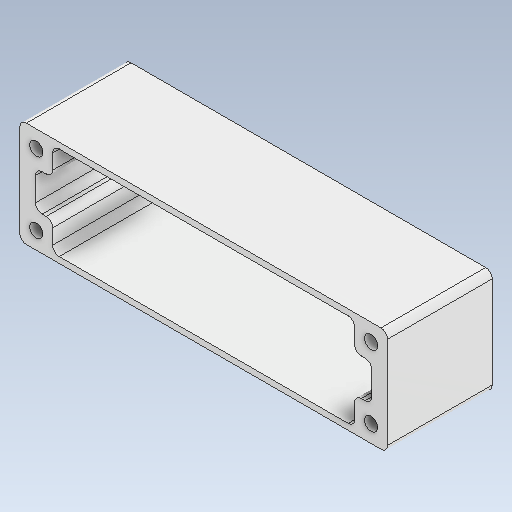
# Autodesk Inventor part: Battery Holder
Saved by Autodesk Inventor 2020 (Build 240168000, 168)
## iProperties
Created: 2020-02-03
Part Number: Battery Holder
Material: PC/ABS Plastic
Document SubType Name: Modeling
Designer: GJCla
Density: 0.357273 g/cm^3
Appearance: Smooth - White
Author: GJCla
Autodesk Inventor part; units mm, degrees
ref_plane "YZ Plane" through (0, 0, 0) normal (1, 0, 0) x (0, 1, 0)
ref_plane "XZ Plane" through (0, 0, 0) normal (0, 1, 0) x (-1, 0, 0)
sketch "Sketch1" plane through (0, 0, 0) normal (0, 0, 1) x (1, 0, 0)
  arc A0 (68.5, 19.5) -> (65.5, 22.5) centre (65.5, 19.5) ccw projected
  line L0 (-65.5, 22.5) -> (65.5, 22.5) projected
  arc A1 (-65.5, 22.5) -> (-68.5, 19.5) centre (-65.5, 19.5) ccw projected
  line L1 (-68.5, -19.5) -> (-68.5, 19.5) projected
  arc A2 (-68.5, -19.5) -> (-65.5, -22.5) centre (-65.5, -19.5) ccw projected
  line L2 (65.5, -22.5) -> (-65.5, -22.5) projected
  arc A3 (65.5, -22.5) -> (68.5, -19.5) centre (65.5, -19.5) ccw projected
  line L3 (68.5, 19.5) -> (68.5, -19.5) projected
  line L4 (88.6498, -25.3956) -> (-89.1502, -25.3956)
  line L5 (-89.1502, -25.3956) -> (-89.1502, 25.4044)
  line L6 (-89.1502, 25.4044) -> (88.6498, 25.4044)
  line L7 (88.6498, 25.4044) -> (88.6498, -25.3956)
  line L8 (-0.2502, 266.6127) -> (-0.2502, -243.9407)
  point P0 (0, 0)
  dimension "d23" = 177.8
  dimension "d24" = 50.8
  constraints: 10 end point, 2 horizontal, 2 parallel, 1 perpendicular, 1 vertical, 3 other
  measures "d23" distance of L5.end L6.end
  measures "d24" distance of L4.end L5.end
ref_plane "Work Plane1" through (-104.8982, -25.3956, -49) normal (0, 0, 1) x (1, 0, 0)
extrude "Extrusion1" add sketch "Sketch1" against normal up to surface (49 mm away) contours A0 L0 L8 L6 L7 L4 L2 A3 L3 | L0 A1 L1 A2 L2 L8 L4 L5 L6
sketch "Sketch2" plane through (0, 0, 0) normal (0, 0, 1) x (1, 0, 0)
  line L0 (88.6498, -25.3956) -> (88.6498, 25.4044) projected
  line L1 (-89.1502, 25.4044) -> (-89.1502, -25.3956) projected
  arc A0 (68.5, 19.5) -> (65.5, 22.5) centre (65.5, 19.5) ccw projected
  line L2 (68.5, 19.5) -> (68.5, -19.5) projected
  arc A1 (65.5, -22.5) -> (68.5, -19.5) centre (65.5, -19.5) ccw projected
  line L3 (65.5, -22.5) -> (-65.5, -22.5) projected
  arc A2 (-68.5, -19.5) -> (-65.5, -22.5) centre (-65.5, -19.5) ccw projected
  line L4 (-68.5, -19.5) -> (-68.5, 19.5) projected
  arc A3 (-65.5, 22.5) -> (-68.5, 19.5) centre (-65.5, 19.5) ccw projected
  line L5 (-65.5, 22.5) -> (65.5, 22.5) projected
  line L6 (65.5, 22.5) -> (-65.5, 22.5) projected
  line L7 (-65.5, 22.5) -> (-73.2752, 22.5)
  line L8 (-73.2752, 22.5) -> (-73.2752, 8.8856)
  line L9 (-73.2752, 8.8856) -> (-81.5302, 8.8856)
  line L10 (-81.5302, 8.8856) -> (-81.5302, -8.8944)
  line L11 (-81.5302, -8.8944) -> (-73.2752, -8.8944)
  line L12 (-73.2752, -8.8944) -> (-73.2752, -22.5088)
  line L13 (-73.2752, -22.5088) -> (72.7748, -22.5088)
  line L14 (72.7748, -22.5088) -> (72.7748, -8.8944)
  line L15 (72.7748, -8.8944) -> (81.0298, -8.8944)
  line L16 (81.0298, -8.8944) -> (81.0298, 8.8856)
  line L17 (81.0298, 8.8856) -> (72.7748, 8.8856)
  line L18 (72.7748, 8.8856) -> (72.7748, 22.5)
  line L19 (-65.5, 22.5) -> (72.7748, 22.5)
  line L20 (88.6498, 25.4044) -> (-89.1502, 25.4044) projected
  line L21 (-89.1502, -25.3956) -> (88.6498, -25.3956) projected
  point P0 (0, 0)
  dimension "d4" = 45.0088
  dimension "d5" = 17.78
  dimension "d6" = 7.62
  dimension "d7" = 7.62
  dimension "d8" = 146.05
  constraints: 26 end point, 8 perpendicular, 7 point on line, 3 collinear, 1 horizontal
  measures "d4" distance between parallel lines of L13 L6
  measures "d5" distance between parallel lines of L9 L11
  measures "d6" distance between parallel lines of L1 L10
  measures "d7" distance between parallel lines of L0 L16
  measures "d8" distance between parallel lines of L18 L8
extrude "Extrusion2" cut sketch "Sketch2" against normal up to next contours A0 L19 L18 L17 L16 L15 L14 L13 L12 L11 L10 L9 L8 L7 A3 L4 A2 L3 A1 L2
sketch "Sketch5" plane through (88.6498, 25.4044, -49) normal (0, 0, -1) x (-1, 0, 0)
  line L0 (0, 0) -> (0, -50.8) projected
  line L1 (177.8, -50.8) -> (0, -50.8) projected
  line L2 (0, 0) -> (177.8, 0)
  line L3 (177.8, 0) -> (177.8, -50.8)
  line L4 (177.8, -50.8) -> (0, -50.8)
  line L5 (0, -50.8) -> (0, 0)
  point P0 (88.6498, -25.4044)
  constraints: 8 end point, 2 parallel, 1 horizontal, 1 perpendicular
fillet "Fillet2" radius 3.175 12 edges at (-73.2752, 8.8856, -24.5) (-73.2752, 22.5, -24.5) (-81.5302, 8.8856, -24.5) (-81.5302, -8.8944, -24.5) (-73.2752, -8.8944, -24.5) (-73.2752, -22.5088, -24.5) (72.7748, -22.5088, -24.5) (72.7748, -8.8944, -24.5) (81.0298, -8.8944, -24.5) (81.0298, 8.8856, -24.5) (72.7748, 8.8856, -24.5) (72.7748, 22.5, -24.5)
sketch "Sketch6" plane through (0, 0, 0) normal (0, 0, 1) x (1, 0, 0)
  line L0 (-89.1502, 25.4044) -> (-89.1502, -25.3956) projected
  line L1 (-89.1502, -25.3956) -> (88.6498, -25.3956) projected
  line L2 (88.6498, 25.4044) -> (-89.1502, 25.4044) projected
  line L3 (88.6498, -25.3956) -> (88.6498, 25.4044) projected
  point P0 (0, 0)
  point P1 (-81.2127, 17.1494)
  point P2 (-81.2127, -17.1406)
  point P3 (80.6996, -17.1406)
  point P4 (80.6996, 17.1494)
  dimension "d26" = 7.9375
  dimension "d27" = 8.255
  dimension "d28" = 8.255
  dimension "d29" = 7.9502
  constraints: 2 horizontal alignment, 2 vertical alignment
  measures "d26" distance from line of L0 point (-81.213, 17.149)
  measures "d27" distance from line of L1 point (-81.213, -17.141)
  measures "d28" distance from line of L2 point (-81.213, 17.149)
  measures "d29" distance from line of L3 point (80.7, 17.149)
extrude "Extrusion3" add sketch "Sketch5" along normal blind 1.5875
hole "Hole2" at (-81.2127, 17.1494, 0) at (-81.2127, -17.1406, 0) at (80.6996, -17.1406, 0) at (80.6996, 17.1494, 0) direction (0, 0, -1) diameter 6.35 end through all
fillet "Fillet3" radius 3.175 4 edges at (-89.1502, 25.4044, -25.2938) (-89.1502, -25.3956, -25.2938) (88.6498, 25.4044, -25.2938) (88.6498, -25.3956, -25.2938)
body "Solid1"
